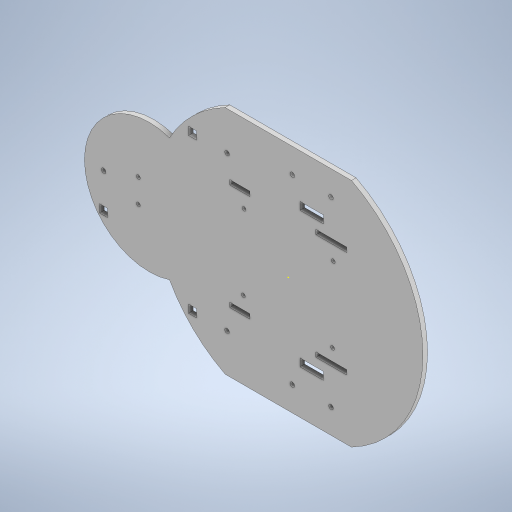
# Autodesk Inventor part: Base component
Saved by Autodesk Inventor 2023 (Build 270158000, 158)
## iProperties
Created: 2023-09-28
Part Number: Base component
Material: Generic
Document SubType Name: Modeling
Designer: say514
Density: 1 g/cm^3
Appearance: Default
Author: say514
Autodesk Inventor part; units mm, degrees
ref_plane "YZ Plane" through (0, 0, 0) normal (1, 0, 0) x (0, 1, 0)
ref_plane "XZ Plane" through (0, 0, 0) normal (0, 1, 0) x (-1, 0, 0)
ref_plane "XY Plane" through (0, 0, 0) normal (0, 0, 1) x (1, 0, 0)
sketch "Base" plane through (0, 0, 0) normal (0, 0, 1) x (1, 0, 0)
  circle A0 centre (-28.7523, 24.2466) radius 1.25 projected
  circle A1 centre (-29.1949, -24.7514) radius 1.25 projected
  arc A2 (-77.2059, 40) -> (-77.2059, -40) centre (-90.3849, 0) ccw
  line L0 (41.0629, -75.0587) -> (-41.0629, -75.0587)
  ellipse E0 centre (0, 0) end of major axis (-87.5, 0) minor radius 85 (-77.2059, -40) -> (-41.0629, -75.0587) ccw
  line L1 (0, 0) -> (87.5, 0)
  line L2 (41.0629, 75.0587) -> (-41.0629, 75.0587)
  ellipse E1 centre (0, 0) end of major axis (-87.5, 0) minor radius 85 (41.0629, -75.0587) -> (41.0629, 75.0587) ccw
  ellipse E2 centre (0, 0) end of major axis (-87.5, 0) minor radius 85 (-41.0629, 75.0587) -> (-77.2059, 40) ccw
  circle A3 centre (29.2453, 23.7226) radius 1.25 projected
  circle A4 centre (28.8027, -25.2754) radius 1.25 projected
  dimension "d84" = 87.5
  dimension "d85" = 75.0587
  dimension "d88" = 42.1151
  constraints: 6 end point, 4 horizontal, 2 point on circle, 2 symmetric about line, 1 centre point, 12 other
  measures "d84" distance of L1.end L1.start
  measures "d85" distance between parallel lines of L1 L2
  measures "d88" radius of A2
sketch "Holes and Mounts" plane through (0, 0, 0) normal (0, 0, 1) x (1, 0, 0)
  line L0 (-9.7798, -74.0877) -> (40.2202, -74.0877)
  circle A0 centre (2.62, -59.0877) radius 1.5
  circle A1 centre (27.82, -59.0877) radius 1.5
  circle A2 centre (-39.757, 45.9313) radius 1.5
  line L1 (-59.657, 43.3313) -> (-64.857, 43.3313)
  line L2 (-64.857, 43.3313) -> (-64.857, 48.5313)
  line L3 (-64.857, 48.5313) -> (-59.657, 48.5313)
  line L4 (-59.657, 48.5313) -> (-59.657, 43.3313)
  line L5 (-59.657, 43.3313) -> (-64.857, 48.5313) construction
  line L6 (-64.857, 43.3313) -> (-59.657, 48.5313) construction
  line L7 (-9.7798, -74.0877) -> (-9.7798, -44.0877)
  line L8 (-9.7798, -44.0877) -> (40.2202, -44.0877)
  line L9 (40.2202, -44.0877) -> (40.2202, -74.0877)
  line L10 (59.2442, -0.0127) -> (-26.2941, -0.0127)
  circle A3 centre (2.62, 59.0622) radius 1.5
  circle A4 centre (27.82, 59.0622) radius 1.5
  line L11 (-9.7798, 74.0622) -> (40.2202, 74.0622)
  line L12 (-9.7798, 44.0622) -> (40.2202, 44.0622)
  line L13 (40.2202, 74.0622) -> (40.2202, 44.0622)
  line L14 (-9.7798, 74.0622) -> (-9.7798, 44.0622)
  circle A5 centre (-39.757, -45.9568) radius 1.5
  line L15 (-59.657, -48.5568) -> (-59.657, -43.3568)
  line L16 (-64.857, -48.5568) -> (-59.657, -48.5568)
  line L17 (-59.657, -43.3568) -> (-64.857, -43.3568)
  line L18 (-64.857, -43.3568) -> (-64.857, -48.5568)
  line L19 (-59.657, -43.3568) -> (-64.857, -48.5568) construction
  line L20 (-64.857, -43.3568) -> (-59.657, -48.5568) construction
  dimension "d53" = 3
  dimension "d54" = 5.2
  dimension "d55" = 5.2
  dimension "d62" = 30
  constraints: 42 end point, 11 symmetric about line, 6 centre point, 3 parallel, 3 perpendicular, 2 horizontal, 1 vertical, 3 other
  measures "d53" diameter of A2
  measures "d54" distance of L3.start L4.start
  measures "d55" distance of L1.end L3.start
  measures "d62" distance of L0.start L7.end
extrude "ComponentARBHoles" add sketch "Base" along normal blind 3
sketch "Holes Only" plane through (0, 0, 3) normal (0, 0, 1) x (1, 0, 0)
  line L0 (-117.446, -25.0998) -> (-117.446, -19.8998)
  line L1 (-117.446, -19.8998) -> (-122.646, -19.8998)
  line L2 (-122.646, -19.8998) -> (-122.646, -25.0998)
  circle A0 centre (-120.046, 0.0002) radius 1.5
  line L3 (-122.646, -25.0998) -> (-117.446, -25.0998)
  circle A1 centre (27.82, -59.0877) radius 1.5
  line L4 (27.82, -59.0877) -> (2.62, -59.0877)
  circle A2 centre (27.82, -59.0877) radius 1.5
  circle A3 centre (2.62, -59.0877) radius 1.5
  circle A4 centre (2.62, -59.0877) radius 1.5
  circle A5 centre (2.62, 59.0622) radius 1.5
  line L5 (2.62, 59.0622) -> (27.82, 59.0622)
  circle A6 centre (2.62, 59.0622) radius 1.5
  circle A7 centre (27.82, 59.0622) radius 1.5
  point P0 (0, 0)
  constraints: 12 end point, 8 centre point, 4 coincident
extrude "WheelFrontSensorHoles" cut sketch "Holes Only" against normal blind 10
sketch "SensorHolesSidesSketch" plane through (0, 0, 0) normal (0, 0, -1) x (-1, 0, 0)
  circle A0 centre (39.757, -50.0587) radius 1.5
  line L0 (64.857, -52.6587) -> (59.657, -52.6587)
  line L1 (64.857, -47.4587) -> (64.857, -52.6587)
  line L2 (59.657, -47.4587) -> (64.857, -47.4587)
  line L3 (59.657, -52.6587) -> (59.657, -47.4587)
  circle A1 centre (39.757, -50.0587) radius 1.5
  line L4 (64.857, -52.6587) -> (59.657, -52.6587)
  line L5 (59.657, -52.6587) -> (59.657, -47.4587)
  line L6 (59.657, -47.4587) -> (64.857, -47.4587)
  line L7 (64.857, -47.4587) -> (64.857, -52.6587)
  line L8 (39.757, -45.9568) -> (39.757, -75.0587)
  line L9 (41.0629, -75.0587) -> (-41.0629, -75.0587) projected
  line L10 (39.757, -75.0587) -> (39.757, -50.0587)
  point P0 (0, 0)
  point P1 (39.757, 45.9313)
  point P2 (59.657, 48.5313)
  constraints: 20 end point, 2 centre point, 2 point on line, 1 coincident, 1 vertical
sketch "Sketch9" plane through (0, 0, 3) normal (0, 0, 1) x (1, 0, 0)
  point P0 (0, 0)
sketch "HolderSlotsSketch" plane through (0, 0, 0) normal (0, 0, -1) x (-1, 0, 0)
  line L0 (-41.0629, 75.0587) -> (41.0629, 75.0587) projected
  line L1 (22.9567, 75.0587) -> (-16.4493, 75.0587)
  line L2 (0, 0) -> (-128.8133, 0)
  line L3 (0, 0) -> (-38, 0)
  line L4 (-38, 33) -> (-38, 36)
  line L5 (-38, 36) -> (-18, 36)
  line L6 (25, 36) -> (38, 36)
  line L7 (38, 36) -> (38, 33)
  line L8 (38, 0) -> (0, 0)
  line L9 (-38, 36) -> (-18, 36)
  line L10 (-18, 36) -> (-18, 33)
  line L11 (-18, 33) -> (-38, 33)
  line L12 (-38, 33) -> (-38, 36)
  line L13 (38, 36) -> (25, 36)
  line L14 (25, 36) -> (25, 33)
  line L15 (25, 33) -> (38, 33)
  line L16 (38, 33) -> (38, 36)
  line L17 (-38, -33) -> (-38, -36)
  line L18 (-38, -36) -> (-18, -36)
  line L19 (25, -36) -> (38, -36)
  line L20 (38, -36) -> (38, -33)
  line L21 (-38, -36) -> (-18, -36)
  line L22 (-18, -36) -> (-18, -33)
  line L23 (-18, -33) -> (-38, -33)
  line L24 (-38, -33) -> (-38, -36)
  line L25 (38, -36) -> (25, -36)
  line L26 (25, -36) -> (25, -33)
  line L27 (25, -33) -> (38, -33)
  line L28 (38, -33) -> (38, -36)
  constraints: 56 end point, 8 symmetric about line, 5 point on line, 4 horizontal, 4 parallel, 4 perpendicular, 1 vertical
extrude "HolderSlots" cut sketch "HolderSlotsSketch" against normal blind 10
sketch "Sketch11" plane through (0, 0, 0) normal (0, 0, -1) x (-1, 0, 0)
  ellipse E0 centre (0, 0) end of major axis (87.5, 0) minor radius 85 (-41.0629, 75.0587) -> (-41.0629, -75.0587) ccw projected
  circle A0 centre (0, 0) radius 81.5
  line L0 (-81.5, 0) -> (-87.5, 0)
  line L1 (-81.5, 0) -> (-84.5, 0)
  circle A1 centre (-84.5, 0) radius 3
  circle A2 centre (-84.5, 0) radius 2
  dimension "d100" = 163
  dimension "d101" = 4
  constraints: 4 end point, 3 coincident, 2 horizontal alignment, 1 centre point, 1 horizontal, 1 midpoint, 6 other
  measures "d101" diameter of A2
extrude "MagnetHoleBottom" cut sketch "Sketch11" against normal blind 1.5 contours A2 L0 | L0 A2
sketch "Sketch13" plane through (0, 0, 0) normal (0, 0, -1) x (-1, 0, 0)
  circle A0 centre (74.8228, 39.4351) radius 2
  circle A1 centre (74.98, -38.7948) radius 2
  circle A2 centre (74.98, -38.7948) radius 2
  circle A3 centre (74.8228, 39.4351) radius 2
  point P0 (0, 0)
  constraints: 4 centre point, 2 coincident
extrude "MagnetHoleSides" cut sketch "Sketch13" against normal blind 1.5
sketch "Sketch14" plane through (0, 0, 0) normal (0, 0, -1) x (-1, 0, 0)
  circle A0 centre (-27.82, 59.0622) radius 1.5 construction
  circle A1 centre (-2.62, 59.0622) radius 1.5 construction
  line L0 (-7.62, 45.0622) -> (-7.62, 41.5622)
  line L1 (-7.62, 41.5622) -> (-22.82, 41.5622)
  line L2 (-22.82, 41.5622) -> (-22.82, 44.0622)
  line L3 (-7.62, 45.0622) -> (-7.62, 46.5622)
  line L4 (-7.62, 46.5622) -> (-22.82, 46.5622)
  line L5 (-22.82, 46.5622) -> (-22.82, 44.0622)
  point P0 (0, 0)
  dimension "d120" = 2.5
  dimension "d121" = 2.5
  constraints: 12 end point, 2 perpendicular, 1 vertical
  measures "d120" distance of L2.end L1.end
  measures "d121" distance of L2.end L4.end
extrude "Extrusion10" cut sketch "Sketch14" against normal blind 10
mirror "Mirror2" about plane through (0, 0, 0) normal (0, 1, 0) of "Extrusion10"
sketch "Sketch15" plane through (0, 0, 0) normal (0, 0, -1) x (-1, 0, 0)
  circle A0 centre (97.5, 7.7) radius 1.27
  circle A1 centre (97.5, -7.7) radius 1.27
  line L0 (-41.4439, -82.7587) -> (-41.4439, -75.0587)
  arc A2 (77.2059, -40) -> (77.2059, 40) centre (90.3849, 0) ccw projected
  point P0 (0, 0)
  dimension "d122" = 2.54
  dimension "d123" = 2.54
  constraints: 2 centre point, 2 end point
  measures "d122" diameter of A0
  measures "d123" diameter of A1
extrude "Ball Caster Holes" cut sketch "Sketch15" against normal blind 10
extrude "Extrusion12" cut sketch "SensorHolesSidesSketch" against normal blind 10
mirror "Mirror3" about plane through (0, 0, 0) normal (0, 1, 0) of "Extrusion12"
body "Solid2"
